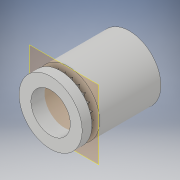
# Autodesk Inventor part: Thoughts for a new driver gear
Saved by Autodesk Inventor 2019 (Build 230136000, 136)
## iProperties
Created: 2021-04-30
Part Number: Thoughts for a new driver gear
Material: Generic
Document SubType Name: Modeling
Designer: Ian
Density: 1 g/cm^3
Appearance: Default
Author: Ian
Autodesk Inventor part; units mm, degrees
ref_plane "YZ Plane" through (0, 0, 0) normal (1, 0, 0) x (0, 1, 0)
ref_plane "XZ Plane" through (0, 0, 0) normal (0, 1, 0) x (-1, 0, 0)
sketch "Sketch1" plane through (0, 0, 0) normal (0, 0, 1) x (1, 0, 0)
  circle A0 centre (0, 0) radius 2.5
  circle A1 centre (0, 0) radius 4
  line L0 (-3.5063, 3.5) -> (5.715, 3.5) construction
  line L1 (-3.4532, 4.1) -> (5.7681, 4.1) construction
  dimension "d0" = 5
  dimension "d1" = 0.6
  dimension "d2" = 0.1
  dimension "d3" = 1
  constraints: 4 end point, 2 centre point, 2 coincident, 2 horizontal, 1 parallel
  measures "d0" diameter of A0
  measures "d1" distance between parallel lines of L0 L1
  measures "d2" distance edge to line of A1 L1
  measures "d3" distance edge to line of A0 L0
extrude "Extrusion1" add sketch "Sketch1" along normal blind 10
sketch "Sketch2" plane through (0, 0, 0) normal (1, 0, 0) x (0, 1, 0)
  line L0 (4, 10) -> (-4, 10) projected
  line L1 (-4, 0) -> (4, 0) projected
  line L2 (4, 10) -> (4, 8.7612)
  line L3 (4, 0) -> (4, 10) projected
  circle A0 centre (3.8, 8.2731) radius 0.3
  line L4 (4, 8.7612) -> (3.25, 8.2731)
  line L5 (3.25, 8.2731) -> (4, 7.785)
  line L6 (2.5, 0) -> (2.5, 10) projected
  line L7 (0, -2) -> (0, 12) projected
  point P0 (0, 0)
  dimension "d6" = 0.6
  dimension "d7" = 0.1
  dimension "d8" = 0.75
  constraints: 6 end point, 2 point on line, 2 tangent, 1 centre point, 1 equal length
  measures "d6" diameter of A0
  measures "d7" distance edge to line of A0 L3
  measures "d8" distance from line of L6 L4.end
revolve "Revolution1" cut sketch "Sketch2" angle 360 about axis through (0, 0, -10) along (0, 0, 1) picked at (3.9033, 8.3516) contours L3 A0 L4 | L3 A0 | A0 L5 L4 | L3 L5 A0
ref_plane "Work Plane1" through (0, 3.25, 8.2731) normal (0, 0, 1) x (1, 0, 0)
sketch "Sketch4" plane through (0, 3.25, 8.2731) normal (0, 0, 1) x (1, 0, 0)
  line L0 (-1.6699, 0.85) -> (1.5938, 0.85) construction
  line L1 (-1.4284, 0.3) -> (1.8353, 0.3) construction
  circle A0 centre (0, -3.25) radius 4 projected
  circle A1 centre (0, -3.25) radius 3.25 projected
  line L2 (0, -3.25) -> (-0.2833, -0.0124)
  line L3 (0, -3.25) -> (0.2833, -0.0124)
  arc A2 (0.2833, -0.0124) -> (-0.2833, -0.0124) centre (0, -3.25) ccw
  line L4 (-0.2833, -0.0124) -> (0, 0.3)
  line L5 (0, 0.3) -> (0.2833, -0.0124)
  point P0 (0, 0)
  dimension "d16" = 0.55
  dimension "d17" = 0.1
  dimension "d18" = 10
  constraints: 12 end point, 5 point on circle, 2 horizontal, 1 centre point, 1 concentric, 1 parallel, 1 point on line, 1 vertical alignment
  measures "d16" distance between parallel lines of L1 L0
  measures "d17" distance edge to line of A0 L0
  measures "d18" angle of L3 L2
extrude "Extrusion3" add sketch "Sketch4" along normal through all both and the other way through all contours A1 L4 L5
sketch "Sketch3" plane through (0, 3.25, 8.2731) normal (0, 0, 1) x (1, 0, 0)
  line L0 (0, -3.25) -> (-0.1745, 0.7462) construction
  circle A0 centre (0, -3.25) radius 4 projected
  line L1 (0, -3.25) -> (0.1745, 0.7462) construction
  arc A1 (0.1745, 0.7462) -> (-0.1745, 0.7462) centre (0, -3.25) ccw
  circle A2 centre (0, -3.25) radius 3.25 projected
  arc A3 (0.1418, -0.0031) -> (-0.1418, -0.0031) centre (0, -3.25) ccw
  line L2 (-0.1745, 0.7462) -> (-0.1418, -0.0031)
  line L3 (0.1418, -0.0031) -> (0.1745, 0.7462)
  line L4 (0, 0.75) -> (-0.1418, -0.0031)
  line L5 (0, 0.75) -> (0.1418, -0.0031)
  point P0 (0, 0)
  dimension "d10" = 5
  constraints: 12 end point, 10 point on circle, 2 centre point, 2 concentric, 2 point on line, 1 collinear, 1 equal length, 1 vertical alignment
  measures "d10" angle of L1 L0
pattern_circular "Circular Pattern2" count 24 over 360 about axis through (0, 0, -10) along (0, 0, 1) of "Extrusion3"
body "Solid1"
